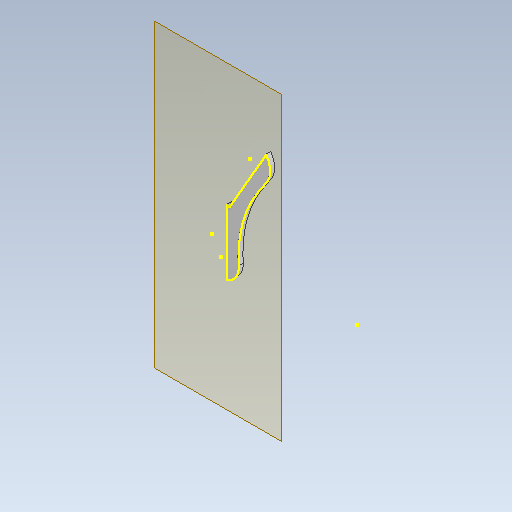
# Autodesk Inventor part: wooden_stiffener
Saved by Autodesk Inventor 2020 (Build 240168000, 168)
## iProperties
Created: 2019-07-26
Part Number: wooden_stiffener
Material: Generic
Document SubType Name: Modeling
Designer: erwin
Density: 1 g/cm^3
Appearance: Default
Author: erwin
Autodesk Inventor part; units mm, degrees
ref_plane "YZ Plane" through (0, 0, 0) normal (1, 0, 0) x (0, 1, 0)
ref_plane "XZ Plane" through (0, 0, 0) normal (0, 1, 0) x (-1, 0, 0)
ref_plane "XY Plane" through (0, 0, 0) normal (0, 0, 1) x (1, 0, 0)
ref_plane "Work Plane1" through (0, 0, 20) normal (0, 0, 1) x (1, 0, 0)
sketch "Sketch1" plane through (0, 0, 20) normal (0, 0, 1) x (1, 0, 0)
  circle A0 centre (68.2595, 214.6541) radius 4 projected
  line L0 (64.2595, -185.3459) -> (64.2595, -225.3459) projected
  arc A1 (72.2595, -185.3459) -> (64.2595, -185.3459) centre (68.2595, -185.3459) ccw projected
  line L1 (72.2595, -225.3459) -> (72.2595, -185.3459) projected
  arc A2 (64.2595, -225.3459) -> (72.2595, -225.3459) centre (68.2595, -225.3459) ccw projected
  line L2 (-101.2595, 230.5421) -> (-90.8671, 224.5421) projected
  line L3 (-90.8671, 224.5421) -> (-108.8671, 193.3652) projected
  line L4 (-108.8671, 193.3652) -> (-119.2595, 199.3652) projected
  line L5 (-137.2595, 168.1883) -> (-119.2595, 199.3652) projected
  line L6 (-137.2595, 168.1883) -> (-106.0825, 150.1883) projected
  line L7 (-106.0825, 150.1883) -> (-112.0825, 139.796) projected
  line L8 (-80.9056, 121.796) -> (-112.0825, 139.796) projected
  line L9 (-80.9056, 121.796) -> (-74.9056, 132.1883) projected
  line L10 (-74.9056, 132.1883) -> (-43.7287, 114.1883) projected
  line L11 (-43.7287, 114.1883) -> (-49.7287, 103.796) projected
  line L12 (-18.5518, 85.796) -> (-49.7287, 103.796) projected
  line L13 (-18.5518, 85.796) -> (-12.5518, 96.1883) projected
  line L14 (-12.5518, 96.1883) -> (18.6251, 78.1883) projected
  line L15 (18.6251, 78.1883) -> (12.6251, 67.796) projected
  line L16 (23.2595, 61.6562) -> (12.6251, 67.796) projected
  line L17 (23.2595, -7.001) -> (23.2595, 61.6562) projected
  line L18 (23.2595, -7.001) -> (35.2595, -7.001) projected
  line L19 (35.2595, -7.001) -> (35.2595, -43.001) projected
  line L20 (35.2595, -43.001) -> (23.2595, -43.001) projected
  line L21 (23.2595, -79.001) -> (23.2595, -43.001) projected
  line L22 (23.2595, -79.001) -> (35.2595, -79.001) projected
  line L23 (35.2595, -79.001) -> (35.2595, -115.001) projected
  line L24 (35.2595, -115.001) -> (23.2595, -115.001) projected
  line L25 (23.2595, -151.001) -> (23.2595, -115.001) projected
  line L26 (23.2595, -151.001) -> (35.2595, -151.001) projected
  line L27 (35.2595, -151.001) -> (35.2595, -187.001) projected
  line L28 (35.2595, -187.001) -> (23.2595, -187.001) projected
  line L29 (23.2595, -223.001) -> (23.2595, -187.001) projected
  line L30 (23.2595, -223.001) -> (35.2595, -223.001) projected
  line L31 (35.2595, -223.001) -> (35.2595, -259.001) projected
  line L32 (35.2595, -259.001) -> (23.2595, -259.001) projected
  line L33 (23.2595, -295.001) -> (23.2595, -259.001) projected
  line L34 (23.2595, -295.001) -> (35.2595, -295.001) projected
  line L35 (35.2595, -295.001) -> (35.2595, -331.001) projected
  line L36 (105.7595, -290.2979) -> (35.2595, -331.001) projected
  arc A3 (105.7595, -290.2979) -> (143.2595, -225.3459) centre (68.2595, -225.3459) ccw projected
  line L37 (143.2595, -185.3459) -> (143.2595, -225.3459) projected
  arc A4 (143.2595, -185.3459) -> (125.3012, -136.6505) centre (68.2595, -185.3459) ccw projected
  arc A5 (114.6586, -107.7924) -> (125.3012, -136.6505) centre (159.1055, -107.7924) ccw projected
  line L38 (114.6586, 129.2663) -> (114.6586, -107.7924) projected
  arc A6 (5.9066, 302.615) -> (62.9654, 289.467) centre (55.9066, 389.2175) ccw projected
  line L39 (-43.2595, 331.001) -> (5.9066, 302.615) projected
  line L40 (-65.2595, 292.8959) -> (-43.2595, 331.001) projected
  line L41 (-65.2595, 292.8959) -> (-54.8671, 286.8959) projected
  line L42 (-54.8671, 286.8959) -> (-72.8671, 255.719) projected
  line L43 (-72.8671, 255.719) -> (-83.2595, 261.719) projected
  line L44 (-101.2595, 230.5421) -> (-83.2595, 261.719) projected
  circle A7 centre (28.2595, 174.6541) radius 30 projected
  line L45 (71.9456, 130.5421) -> (61.5533, 136.5421) projected
  line L46 (61.5533, 136.5421) -> (79.5533, 167.719) projected
  line L47 (79.5533, 167.719) -> (89.9456, 161.719) projected
  line L48 (89.9456, 161.719) -> (71.9456, 130.5421) projected
  line L49 (40.4552, 75.9992) -> (71.9456, 130.5421) projected
  line L50 (40.4552, 75.9992) -> (30.0629, 81.9992) projected
  line L51 (30.0629, 81.9992) -> (61.5533, 136.5421) projected
  line L52 (61.5533, 136.5421) -> (71.9456, 130.5421) projected
  line L53 (40.4552, 75.9992) -> (71.9456, 130.5421) projected
  line L54 (35.2595, 78.999) -> (35.2595, -6.251) projected
  line L55 (35.2595, -6.251) -> (23.2595, -6.251) projected
  line L56 (23.2595, 78.999) -> (23.2595, -6.251) projected
  line L57 (35.2595, 78.999) -> (23.2595, 78.999) projected
  line L58 (89.9456, 161.719) -> (137.3521, 243.8295)
  line L59 (131.6514, 174.8386) -> (110.2726, 142.3196)
  arc A8 (110.2726, 142.3196) -> (63.3739, -36.5254) centre (352.1075, -16.6687) ccw
  arc A9 (35.2595, -79.001) -> (63.3739, -36.5254) centre (21.5733, -39.4001) ccw
  line L60 (119.5533, 237.001) -> (129.9456, 231.001) projected
  arc A10 (131.6514, 174.8386) -> (129.9456, 231.001) centre (90.7859, 201.7046) ccw
  circle A11 centre (68.2595, 214.6541) radius 4 projected
  line L61 (64.2595, -185.3459) -> (64.2595, -225.3459) projected
  arc A12 (72.2595, -185.3459) -> (64.2595, -185.3459) centre (68.2595, -185.3459) ccw projected
  line L62 (72.2595, -225.3459) -> (72.2595, -185.3459) projected
  arc A13 (64.2595, -225.3459) -> (72.2595, -225.3459) centre (68.2595, -225.3459) ccw projected
  line L63 (-101.2595, 230.5421) -> (-90.8671, 224.5421) projected
  line L64 (-90.8671, 224.5421) -> (-108.8671, 193.3652) projected
  line L65 (-108.8671, 193.3652) -> (-119.2595, 199.3652) projected
  line L66 (-137.2595, 168.1883) -> (-119.2595, 199.3652) projected
  line L67 (-137.2595, 168.1883) -> (-106.0825, 150.1883) projected
  line L68 (-106.0825, 150.1883) -> (-112.0825, 139.796) projected
  line L69 (-80.9056, 121.796) -> (-112.0825, 139.796) projected
  line L70 (-80.9056, 121.796) -> (-74.9056, 132.1883) projected
  line L71 (-74.9056, 132.1883) -> (-43.7287, 114.1883) projected
  line L72 (-43.7287, 114.1883) -> (-49.7287, 103.796) projected
  line L73 (-18.5518, 85.796) -> (-49.7287, 103.796) projected
  line L74 (-18.5518, 85.796) -> (-12.5518, 96.1883) projected
  line L75 (-12.5518, 96.1883) -> (18.6251, 78.1883) projected
  line L76 (18.6251, 78.1883) -> (12.6251, 67.796) projected
  line L77 (23.2595, 61.6562) -> (12.6251, 67.796) projected
  line L78 (23.2595, -7.001) -> (23.2595, 61.6562) projected
  line L79 (23.2595, -7.001) -> (35.2595, -7.001) projected
  line L80 (35.2595, -7.001) -> (35.2595, -43.001) projected
  line L81 (35.2595, -43.001) -> (23.2595, -43.001) projected
  line L82 (23.2595, -79.001) -> (23.2595, -43.001) projected
  line L83 (23.2595, -79.001) -> (35.2595, -79.001) projected
  line L84 (35.2595, -79.001) -> (35.2595, -115.001) projected
  line L85 (35.2595, -115.001) -> (23.2595, -115.001) projected
  line L86 (23.2595, -151.001) -> (23.2595, -115.001) projected
  line L87 (23.2595, -151.001) -> (35.2595, -151.001) projected
  line L88 (35.2595, -151.001) -> (35.2595, -187.001) projected
  line L89 (35.2595, -187.001) -> (23.2595, -187.001) projected
  line L90 (23.2595, -223.001) -> (23.2595, -187.001) projected
  line L91 (23.2595, -223.001) -> (35.2595, -223.001) projected
  line L92 (35.2595, -223.001) -> (35.2595, -259.001) projected
  line L93 (35.2595, -259.001) -> (23.2595, -259.001) projected
  line L94 (23.2595, -295.001) -> (23.2595, -259.001) projected
  line L95 (23.2595, -295.001) -> (35.2595, -295.001) projected
  line L96 (35.2595, -295.001) -> (35.2595, -331.001) projected
  line L97 (105.7595, -290.2979) -> (35.2595, -331.001) projected
  arc A14 (105.7595, -290.2979) -> (143.2595, -225.3459) centre (68.2595, -225.3459) ccw projected
  line L98 (143.2595, -185.3459) -> (143.2595, -225.3459) projected
  arc A15 (143.2595, -185.3459) -> (125.3012, -136.6505) centre (68.2595, -185.3459) ccw projected
  arc A16 (114.6586, -107.7924) -> (125.3012, -136.6505) centre (159.1055, -107.7924) ccw projected
  line L99 (114.6586, 129.2663) -> (114.6586, -107.7924) projected
  arc A17 (128.1281, 169.4795) -> (114.6586, 129.2663) centre (181.4216, 129.2663) ccw projected
  arc A18 (128.1281, 169.4795) -> (62.9654, 289.467) centre (68.2595, 214.6541) ccw projected
  arc A19 (5.9066, 302.615) -> (62.9654, 289.467) centre (55.9066, 389.2175) ccw projected
  line L100 (-43.2595, 331.001) -> (5.9066, 302.615) projected
  line L101 (-65.2595, 292.8959) -> (-43.2595, 331.001) projected
  line L102 (-65.2595, 292.8959) -> (-54.8671, 286.8959) projected
  line L103 (-54.8671, 286.8959) -> (-72.8671, 255.719) projected
  line L104 (-72.8671, 255.719) -> (-83.2595, 261.719) projected
  line L105 (-101.2595, 230.5421) -> (-83.2595, 261.719) projected
  circle A20 centre (28.2595, 174.6541) radius 30 projected
  line L106 (71.9456, 130.5421) -> (61.5533, 136.5421) projected
  line L107 (61.5533, 136.5421) -> (79.5533, 167.719) projected
  line L108 (79.5533, 167.719) -> (89.9456, 161.719) projected
  line L109 (89.9456, 161.719) -> (71.9456, 130.5421) projected
  line L110 (35.2595, -7.001) -> (35.2595, 3.1632)
  line L111 (35.2595, -6.251) -> (35.2595, -79.001)
  point P0 (0, 0)
  constraints: 8 end point, 6 point on circle, 4 point on line, 3 centre point, 3 tangent, 1 collinear
extrude "Extrusion1" add sketch "Sketch1" along normal blind 12 contours A10 L59 A17 A8 A9 L111 L19 L110 L54 L50 L49 L48 L58 | L59 A17
sketch "Sketch3" plane through (0, 0, 32) normal (0, 0, 1) x (1, 0, 0)
  line L0 (35.2595, 78.999) -> (35.2595, -79.001) projected
  arc A0 (35.2595, -79.001) -> (63.3739, -36.5254) centre (21.5733, -39.4001) ccw projected
  arc A1 (110.2726, 142.3196) -> (63.3739, -36.5254) centre (352.1075, -16.6687) ccw projected
  line L1 (110.2726, 142.3196) -> (131.6514, 174.8386) projected
  arc A2 (131.6514, 174.8386) -> (129.9456, 231.001) centre (90.7859, 201.7046) ccw projected
  line L2 (129.9456, 231.001) -> (40.4552, 75.9992) projected
  line L3 (40.4552, 75.9992) -> (35.2595, 78.999) projected
  point P0 (0, 0)
body "Solid1"
